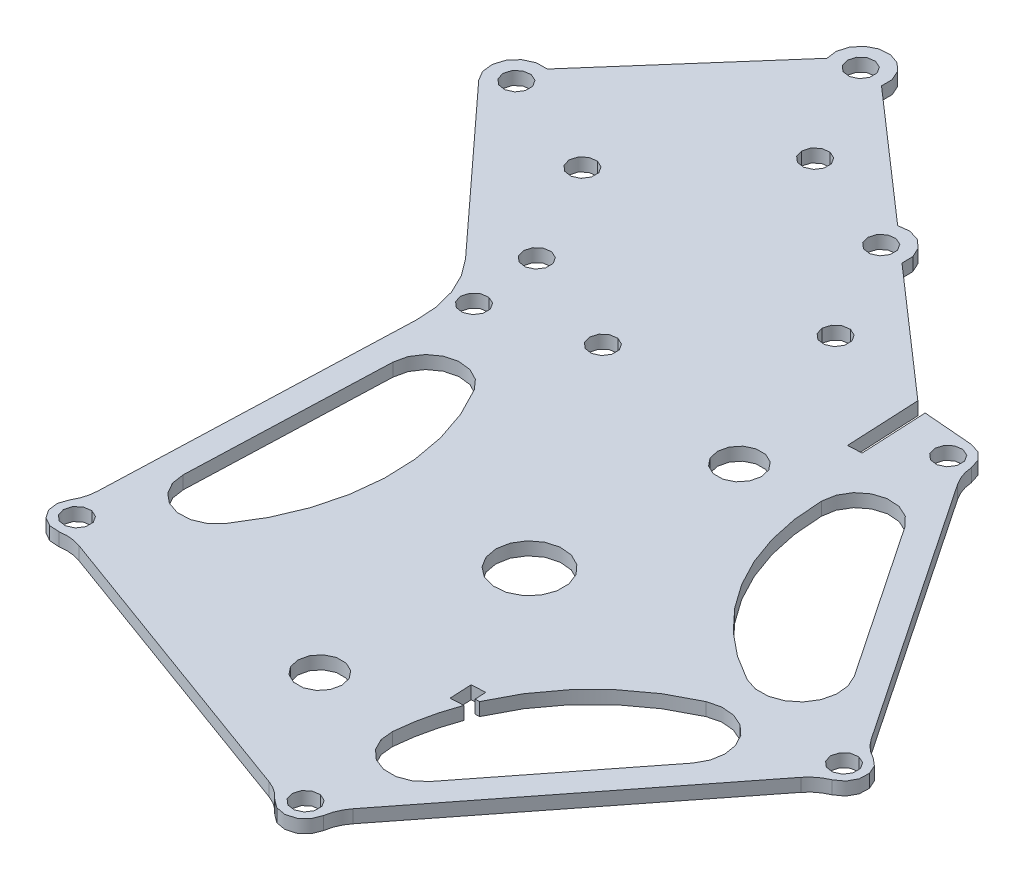
# Autodesk Inventor part: femur_motor_steel
Saved by Autodesk Inventor 2026 (Build 300175000, 175)
## iProperties
Created: 2026-04-24
Part Number: femur_motor_steel
Material: Сталь
Document SubType Name: Modeling
Designer: user
Density: 7.85 g/cm^3
Appearance: Серо-синий
Author: user
Autodesk Inventor part; units mm, degrees
ref_plane "YZ Plane" through (0, 0, 0) normal (1, 0, 0) x (0, 1, 0)
ref_plane "XZ Plane" through (0, 0, 0) normal (0, 1, 0) x (-1, 0, 0)
ref_plane "XY Plane" through (0, 0, 0) normal (0, 0, 1) x (1, 0, 0)
sketch "Эскиз1" plane through (0, 0, 0) normal (0, 1, 0) x (-1, 0, 0)
  circle A0 centre (-104.4495, 228.5917) radius 3.05
  circle A1 centre (-187.2645, 258.8445) radius 3.05
  circle A2 centre (-241.6278, 189.4314) radius 3.05
  circle A3 centre (-192.4112, 116.2789) radius 3.05
  circle A4 centre (-107.6303, 140.4814) radius 3.05
  line L0 (-177.9345, 108.7439) -> (-148.7066, 83.1689) projected
  arc A5 (-148.7066, 83.1689) -> (-140.7553, 76.2113) centre (-142.7225, 81.9854) ccw projected
  line L1 (-140.7553, 76.2113) -> (-111.0782, 50.2432) projected
  arc A6 (-111.0782, 50.2432) -> (-99.32, 51.0269) centre (-105.0941, 49.0597) ccw projected
  line L2 (-99.32, 51.0269) -> (-69.3349, 85.2947) projected
  arc A7 (-69.3349, 85.2947) -> (-63.6584, 95.4047) centre (-68.1514, 91.2788) ccw projected
  line L3 (-63.6584, 95.4047) -> (-126.3351, 163.6585) projected
  arc A8 (-134.2087, 185.2821) -> (-126.3351, 163.6585) centre (-104.2383, 183.9497) ccw projected
  arc A9 (-134.2087, 185.2821) -> (-136.8853, 199.7151) centre (-166.6767, 186.7256) ccw projected
  line L4 (-136.8853, 199.7151) -> (-152.7923, 236.1975) projected
  arc A10 (-152.7923, 236.1975) -> (-173.078, 237.7086) centre (-163.3338, 231.6012) ccw projected
  line L5 (-173.078, 237.7086) -> (-183.3611, 221.3023) projected
  line L6 (-183.3611, 221.3023) -> (-183.1353, 216.6186) projected
  line L7 (-183.1353, 216.6186) -> (-186.3952, 216.4614) projected
  line L8 (-186.3952, 216.4614) -> (-194.2147, 203.9856) projected
  arc A11 (-194.2147, 203.9856) -> (-196.468, 173.7361) centre (-166.6767, 186.7256) ccw projected
  line L9 (-196.468, 173.7361) -> (-188.1074, 154.5612) projected
  arc A12 (-185.6419, 144.0156) -> (-188.1074, 154.5612) centre (-215.6071, 142.5709) ccw projected
  line L10 (-185.6419, 144.0156) -> (-184.8431, 127.4459) projected
  arc A13 (-184.8431, 127.4459) -> (-182.7485, 125.5315) centre (-182.8448, 127.5292) ccw projected
  line L11 (-182.7485, 125.5315) -> (-178.7531, 125.7242) projected
  line L12 (-178.7531, 125.7242) -> (-177.9345, 108.7439) projected
  circle A14 centre (-117.9158, 72.371) radius 3.05 projected
  circle A15 centre (-155.5442, 105.2966) radius 3.05 projected
  circle A16 centre (-130.5866, 133.819) radius 3.05 projected
  circle A17 centre (-105.7799, 124.2045) radius 3.05 projected
  circle A18 centre (-92.9581, 100.8933) radius 3.05 projected
  circle A19 centre (-166.6767, 186.7256) radius 7.75 projected
  circle A20 centre (-163.3338, 231.6012) radius 5.05 projected
  circle A21 centre (-170.0195, 141.8499) radius 5.05 projected
  circle A22 centre (-105.0941, 49.0597) radius 3.05 projected
  circle A23 centre (-142.7225, 81.9854) radius 3.05 projected
  circle A24 centre (-68.1514, 91.2788) radius 3.05 projected
  line L13 (-181.9494, 125.5701) -> (-181.2156, 110.3492)
  line L14 (-186.4116, 221.5666) -> (-183.3809, 221.7127)
  line L15 (-183.3809, 221.7127) -> (-183.3611, 221.3023)
  arc A25 (-183.4563, 262.0845) -> (-192.2092, 259.5858) centre (-187.2645, 258.8445) ccw
  arc A26 (-100.1912, 225.9712) -> (-105.2725, 233.5236) centre (-104.4495, 228.5917) ccw
  arc A27 (-197.3965, 115.8961) -> (-192.7301, 111.2891) centre (-192.4112, 116.2789) ccw
  arc A28 (-243.5325, 194.0544) -> (-243.8609, 184.9577) centre (-241.6278, 189.4314) ccw
  line L16 (-181.2156, 110.3492) -> (-192.8177, 111.2955)
  line L17 (-201.4914, 135.239) -> (-225.4661, 170.8734)
  line L18 (-224.17, 206.7756) -> (-197.6882, 240.5885)
  line L19 (-108.2479, 207.9155) -> (-109.9279, 161.3777)
  circle A29 centre (-166.6767, 186.7256) radius 85 construction
  arc A30 (-122.7619, 212.8408) -> (-129.5158, 167.7928) centre (-81.732, 183.659) ccw
  arc A31 (-213.4906, 192.975) -> (-187.4434, 219.0115) centre (-233.5959, 239.1357) ccw
  arc A32 (-186.8543, 139.7855) -> (-213.8194, 183.8681) centre (-237.2008, 139.2773) ccw
  arc A33 (-186.4116, 221.5666) -> (-183.417, 234.9984) centre (-233.5959, 239.1357) ccw
  arc A34 (-129.5158, 167.7928) -> (-124.7594, 157.5118) centre (-81.732, 183.659) ccw
  arc A35 (-224.17, 206.7756) -> (-213.4906, 192.975) centre (-217.0845, 201.2263) ccw
  arc A36 (-213.8194, 183.8681) -> (-225.4661, 170.8734) centre (-217.9988, 175.8974) ccw
  arc A37 (-183.417, 234.9984) -> (-197.6882, 240.5885) centre (-191.39, 235.6558) ccw
  arc A38 (-108.2479, 207.9155) -> (-122.7619, 212.8408) centre (-116.2427, 208.2041) ccw
  arc A39 (-124.7594, 157.5118) -> (-109.9279, 161.3777) centre (-117.9227, 161.6663) ccw
  arc A40 (-201.4914, 135.239) -> (-186.8543, 139.7855) centre (-194.8539, 139.7047) ccw
  line L20 (-97.6563, 132.4278) -> (-63.6584, 95.4047)
  arc A41 (-104.2261, 150.2391) -> (-97.6563, 132.4278) centre (-79.2423, 149.3372) ccw
  line L21 (-192.7296, 111.2883) -> (-192.7301, 111.2891)
  line L22 (-199.0702, 120.7126) -> (-240.03, 181.5926)
  line L23 (-239.4689, 197.1346) -> (-194.2259, 254.9025)
  line L24 (-101.6683, 221.0907) -> (-104.2261, 150.2391)
  line L25 (-179.2712, 259.1717) -> (-110.3497, 233.9943)
  line L26 (-76.8164, 221.7444) -> (-72.2795, 220.087)
  arc A42 (-100.1912, 225.9712) -> (-101.6683, 221.0907) centre (-91.6748, 220.73) ccw
  arc A43 (-110.3497, 233.9943) -> (-105.2725, 233.5236) centre (-106.9184, 243.3872) ccw
  arc A44 (-183.4563, 262.0845) -> (-179.2712, 259.1717) centre (-175.8399, 268.5646) ccw
  arc A45 (-194.2259, 254.9025) -> (-192.2092, 259.5858) centre (-202.0987, 261.0684) ccw
  arc A46 (-243.5325, 194.0544) -> (-239.4689, 197.1346) centre (-247.3417, 203.3005) ccw
  arc A47 (-240.03, 181.5926) -> (-243.8609, 184.9577) centre (-248.3269, 176.0104) ccw
  arc A48 (-197.3965, 115.8961) -> (-199.0702, 120.7126) centre (-207.3672, 115.1305) ccw
  line L27 (-186.4544, 219.0115) -> (-187.4434, 219.0115)
  line L28 (-186.3316, 216.4645) -> (-186.4544, 219.0115)
  point P0 (0, 0)
  point P1 (-103.021, 138.2699)
  point P2 (-176.2905, 107.3053)
  point P3 (-197.1534, 117.8636)
  point P4 (-241.9468, 184.4416)
  point P5 (-241.5861, 194.4312)
  point P6 (-182.4965, 260.3499)
  point P7 (-192.1086, 257.6059)
  point P8 (-101.5444, 224.5223)
  point P9 (-107.1244, 232.8161)
  point P10 (-186.4116, 221.5666)
  dimension "d5" = 6.1
  dimension "d8" = 360
  dimension "d13" = 3.2
  dimension "d16" = 10
  dimension "d26" = 170
  dimension "d27" = 9
  dimension "d28" = 8
  dimension "d29" = 8
  dimension "d30" = 8
  dimension "d31" = 25
  dimension "d32" = 10
  dimension "d33" = 10
  dimension "d34" = 10
  dimension "d35" = 10
  constraints: 61 point on circle, 42 tangent, 32 end point, 29 centre point, 14 point on line, 8 equal radius, 6 coincident, 5 parallel, 2 perpendicular, 1 collinear, 1 horizontal, 12 other
  measures "d5" diameter of A0
  measures "d13" distance between parallel lines of L12 L13
  measures "d16" diameter of A25
  measures "d26" diameter of A29
  measures "d27" radius of A35
  measures "d28" radius of A38
  measures "d29" radius of A39
  measures "d30" radius of A40
  measures "d31" radius of A41
  measures "d32" radius of A42
  measures "d33" radius of A46
  measures "d34" radius of A47
  measures "d35" radius of A48
extrude "Выдавливание1" add sketch "Эскиз1" along normal blind 3 contours A4 L3 A39 L19 A38 A30 A8 A9 L4 A10 L5 L15 L14 A33 A37 L18 A35 A31 L27 L28 L7 L8 A11 L9 A12 L10 A13 L11 L13 L16 A27 A48 L22 A47 A28 A46 L23 A45 A25 A44 L25 A43 A26 A42 L24 A41 | A4 L3 A7 L2 A6 L1 A5 L0 L12 L11 A13 L10 A12 L9 A11 L8 L7 L6 L5 A10 L4 A9 A8 A34 A39
equation "\"d5\" = d_main_screw_holes"
equation "\"d2\" = thickness_steel"
equation "\"tolerance_plazma\" = 0.1"
equation "\"thickness_steel\" = 3"
equation "\"d_main_screw_holes\" = 6.1"
equation "\"d_main_shaft\" = 15"
equation "\"thickness_profile_tibea\" = 3"
equation "\"hight_shaft_shift\" = 37"
equation "\"thickness_profile_femur\" = 3"
equation "\"width_shaft_shift\" = 35"
equation "\"width_flattened_surface\" = 12"
equation "\"d22\" = d_main_screw_holes"
equation "\"d23\" = d_main_screw_holes"
equation "\"d25\" = d_main_screw_holes"
